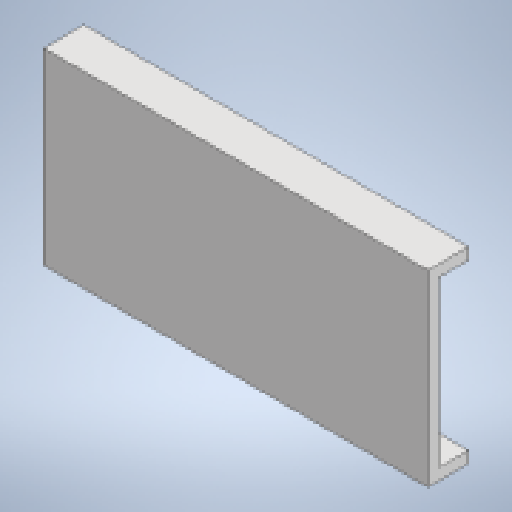
# Autodesk Inventor part: Soporte_ESP32S3
Saved by Autodesk Inventor 2024 (Build 280153000, 153)
## iProperties
Created: 2024-07-20
Part Number: Soporte_ESP32S3
Material: Genérico
Document SubType Name: Modeling
Designer: sergi
Density: 1 g/cm^3
Appearance: Valor por defecto
Author: sergi
Autodesk Inventor part; units mm, degrees
ref_plane "YZ Plane" through (0, 0, 0) normal (1, 0, 0) x (0, 1, 0)
ref_plane "XZ Plane" through (0, 0, 0) normal (0, 1, 0) x (-1, 0, 0)
ref_plane "XY Plane" through (0, 0, 0) normal (0, 0, 1) x (1, 0, 0)
sketch "Boceto1" plane through (0, 0, 0) normal (0, 0, 1) x (1, 0, 0)
  line L0 (-32.25, -14.25) -> (-32.25, 14.25) projected
  line L1 (-32.25, 14.25) -> (32.25, 14.25) projected
  line L2 (32.25, 14.25) -> (32.25, -14.25) projected
  line L3 (32.25, -14.25) -> (-32.25, -14.25) projected
  line L4 (34.25, 16.25) -> (-34.25, 16.25)
  line L5 (-34.25, 16.25) -> (-34.25, -16.25)
  line L6 (-34.25, -16.25) -> (34.25, -16.25)
  line L7 (34.25, -16.25) -> (34.25, 16.25)
  line L8 (32.25, -14.25) -> (32.25, -16.25)
  line L9 (32.25, 14.25) -> (32.25, 16.25)
  point P0 (0, 0)
  dimension "d0" = 2
  constraints: 12 end point, 4 point on line, 3 other
  measures "d0" distance between parallel lines of L1 L4
extrude "Extrusión1" add sketch "Boceto1" along normal blind 2 and the other way blind 5 contours L3 L8 L6 L5 L4 L9 L1 L0 | L0 L1 L2 L3
shell "Vaciado1" thickness 2 removed faces 2 at (32.25, 5.4167, -0.3333) at (-12.0833, 5.4167, -5)
sketch "Boceto2" plane through (0, 0, -5) normal (0, 0, -1) x (-1, 0, 0)
  line L0 (-32.25, 14.25) -> (32.25, 14.25) projected
  line L1 (32.25, 14.25) -> (32.25, -14.25) projected
  line L2 (32.25, -14.25) -> (-32.25, -14.25) projected
  line L3 (-32.25, -14.25) -> (-32.25, -16.25) projected
  line L4 (-32.25, -16.25) -> (34.25, -16.25) projected
  line L5 (34.25, -16.25) -> (34.25, 16.25) projected
  line L6 (34.25, 16.25) -> (-32.25, 16.25) projected
  line L7 (-32.25, 16.25) -> (-32.25, 14.25) projected
  line L8 (-32.25, 16.25) -> (-24.25, 16.25)
  line L9 (-24.25, 16.25) -> (-24.25, 22.25)
  line L10 (-24.25, 22.25) -> (-32.25, 22.25)
  line L11 (-32.25, 22.25) -> (-32.25, 16.25)
  line L12 (-24.25, 22.25) -> (-32.25, 14.25)
  circle A0 centre (-28.25, 18.25) radius 2.1
  point P0 (0, 0)
  point P1 (-30.25, 16.25)
  point P2 (-29.7349, 16.7651)
  point P3 (-27.6097, 16.25)
  point P4 (-28.8903, 16.25)
  dimension "d6" = 8
  dimension "d7" = 6
  dimension "d8" = 4.2
  constraints: 10 end point, 2 parallel, 1 centre point, 1 horizontal, 1 midpoint, 1 perpendicular
  measures "d6" distance of L10.end L9.end
  measures "d7" distance of L9.end L8.end
  measures "d8" diameter of A0
extrude "Extrusión2" add sketch "Boceto2" against normal up to surface (7 mm away) contours L11 L10 L12 A0 L6 | L12 A0 L6 | L9 L6 A0 L12 picked at (-29.8223, 16.5215)
mirror "Simetría1" about plane through (0, 0, 0) normal (0, 1, 0) of "Extrusión2"
ref_plane "Plano de trabajo1" through (-1, -14.25, 0) normal (1, 0, 0) x (0, 0, -1)
mirror "Simetría2" about plane through (-1, -14.25, 0) normal (1, 0, 0) of "Extrusión2", "Simetría1"
fillet "Empalme1" radius 4 12 edges at (-26.25, 22.25, -1.5) (-34.25, 22.25, -1.5) (-34.25, -22.25, -1.5) (-26.25, -22.25, -1.5) (24.25, 22.25, -1.5) (32.25, 22.25, -1.5) (32.25, -22.25, -1.5) (24.25, -22.25, -1.5) (-26.25, 16.25, -1.5) (24.25, 16.25, -1.5) (24.25, -16.25, -1.5) (-26.25, -16.25, -1.5)
sketch "Boceto3" plane through (32.25, -14.25, 0) normal (0, 0, -1) x (-1, 0, 0)
  line L0 (64.5, 0) -> (64.5, 28.5) projected
  line L1 (64.5, 28.5) -> (0, 28.5) projected
  line L2 (0, 28.5) -> (0, 0) projected
  line L3 (0, 0) -> (64.5, 0) projected
  line L4 (64.5, 0) -> (0, 0) projected
  line L5 (0, 28.5) -> (57.5, 28.5)
  line L6 (57.5, 28.5) -> (57.5, 0)
  line L7 (57.5, 0) -> (0, 0)
  line L8 (0, 0) -> (0, 28.5)
  line L9 (54.5, 3) -> (54.5, 25.5)
  line L10 (57.5, 25.5) -> (0, 25.5)
  line L11 (3, 28.5) -> (3, 0)
  line L12 (0, 3) -> (57.5, 3)
  line L13 (2.55, 28.5) -> (2.55, 0)
  point P0 (32.25, 14.25)
  point P1 (57.5, 0)
  point P2 (2.55, 3)
  point P3 (2.55, 0)
  point P4 (2.55, 28.5)
  point P5 (2.55, 25.5)
  dimension "d12" = 57.5
  dimension "d13" = 3
  dimension "d16" = 0.45
  constraints: 18 end point, 9 point on line, 5 parallel, 2 perpendicular, 1 horizontal
  measures "d12" distance of L6.end L7.end
  measures "d13" distance between parallel lines of L6 L9
  measures "d16" distance between parallel lines of L11 L13
extrude "Extrusión3" cut sketch "Boceto3" against normal blind 10 contours L3 L11 L12 L6 | L6 L10 L11 L1 | L3 L13 L12 L11 | L11 L10 L13 L1 | L3 L2 L12 L13 | L13 L10 L2 L1
